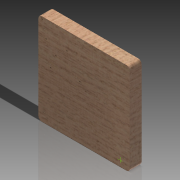
# Autodesk Inventor part: Boden
Saved by Autodesk Inventor 2014 SP1 (Build 180222100, 222)
## iProperties
Created: 2017-12-30
Part Number: Boden
Material: Eiche, weiß
Document SubType Name: Modeling
Designer: Flo
Density: 0.721 g/cm^3
Appearance: Weißeiche - massiv - natur - mittlerer Glanz
Author: Flo
Autodesk Inventor part; units mm, degrees
ref_plane "YZ Plane" through (0, 0, 0) normal (1, 0, 0) x (0, 1, 0)
ref_plane "XZ Plane" through (0, 0, 0) normal (0, 1, 0) x (-1, 0, 0)
ref_plane "XY Plane" through (0, 0, 0) normal (0, 0, 1) x (1, 0, 0)
sketch "Skizze1" plane through (0, 0, 0) normal (0, 1, 0) x (-1, 0, 0)
  line L0 (0, 0) -> (140, 0)
  line L1 (140, 0) -> (140, 140)
  line L2 (140, 140) -> (0, 140)
  line L3 (0, 140) -> (0, 0)
  dimension "d0" = 140
  dimension "d1" = 140
  constraints: 8 end point, 2 parallel, 1 horizontal, 1 perpendicular
  measures "d0" distance of L2.end L1.end
  measures "d1" distance of L1.end L0.end
extrude "Extrusion1" add sketch "Skizze1" along normal blind 18
sketch "Skizze2" plane through (0, 18, 0) normal (0, 1, 0) x (1, 0, 0)
  line L0 (0, 0) -> (-140, 0) projected
  line L1 (-140, 0) -> (-140, -140) projected
  line L2 (-140, -140) -> (0, -140) projected
  line L3 (0, -140) -> (0, 0) projected
  point P0 (-131, -15)
  point P1 (-131, -125)
  point P2 (-9, -15)
  point P3 (-9, -125)
  dimension "d4" = 15
  dimension "d5" = 15
  dimension "d6" = 15
  dimension "d7" = 15
  dimension "d8" = 9
  dimension "d9" = 9
  dimension "d10" = 9
  dimension "d11" = 9
  measures "d4" distance from line of point (-131, -15) L0
  measures "d5" distance from line of L0 point (-9, -15)
  measures "d6" distance from line of L2 point (-131, -125)
  measures "d7" distance from line of L2 point (-9, -125)
  measures "d8" distance from line of L3 point (-9, -125)
  measures "d9" distance from line of L3 point (-9, -15)
  measures "d10" distance from line of L1 point (-131, -15)
  measures "d11" distance from line of L1 point (-131, -125)
hole "Bohrung1" at (-131, 18, 15) at (-131, 18, 125) at (-9, 18, 15) at (-9, 18, 125) direction (0, -1, 0) diameter 2 end through all countersink diameter 5 countersink angle 90
fillet "Rundung1" radius 5 4 edges at (-140, 9, 0) (-140, 9, 140) (0, 9, 140) (0, 9, 0)
sketch "Skizze3" plane through (0, 0, 0) normal (0, -1, 0) x (1, 0, 0)
  point P0 (-15, 9)
